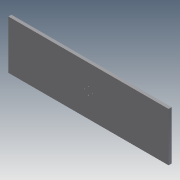
# Autodesk Inventor part: kinect rotate bottom
Saved by Autodesk Inventor 2011 (Build 150239000, 239)
## iProperties
Created: 2012-01-08
Part Number: kinect rotate bottom
Document SubType Name: Modeling
Designer: Matthew
Density: 1 g/cm^3
Author: Matthew
Autodesk Inventor part; units mm, degrees
ref_plane "YZ Plane" through (0, 0, 0) normal (1, 0, 0) x (0, 1, 0)
ref_plane "XZ Plane" through (0, 0, 0) normal (0, 1, 0) x (-1, 0, 0)
ref_plane "XY Plane" through (0, 0, 0) normal (0, 0, 1) x (1, 0, 0)
sketch "Sketch1" plane through (0, 0, 0) normal (0, 0, 1) x (1, 0, 0)
  line L0 (-33.6817, -5.828) -> (300.0743, -5.828)
  line L1 (300.0743, -5.828) -> (300.0743, 7.2749)
  line L2 (300.0743, 7.2749) -> (-33.6817, 7.2749)
  line L3 (-33.6817, 7.2749) -> (-33.6817, -5.828)
  line L4 (-33.6817, 7.2749) -> (300.0743, 7.2749)
  line L5 (300.0743, 7.2749) -> (300.0743, -94.3251)
  line L6 (300.0743, -94.3251) -> (-33.6817, -94.3251)
  line L7 (-33.6817, -94.3251) -> (-33.6817, 7.2749)
  point P0 (0, 0)
  dimension "d0" = 333.756
  dimension "d1" = 101.6
  constraints: 16 end point, 4 parallel, 2 horizontal, 2 perpendicular
  measures "d0" distance of L2.end L1.end
  measures "d1" distance of L4.end L5.end
extrude "Extrusion1" add sketch "Sketch1" along normal blind 6.35
sketch "Sketch2" plane through (0, 0, 6.35) normal (0, 0, 1) x (1, 0, 0)
  circle A0 centre (133.1963, -43.5251) radius 8
  circle A1 centre (133.1963, -35.5251) radius 1
  circle A2 centre (141.1963, -43.5251) radius 1
  circle A3 centre (133.1963, -51.5251) radius 1
  circle A4 centre (125.1963, -43.5251) radius 1
  point P0 (0, 0)
  dimension "d4" = 16
  dimension "d5" = 2
  dimension "d6" = 2
  dimension "d7" = 2
  dimension "d8" = 2
  constraints: 5 centre point, 4 point on circle
  measures "d4" diameter of A0
  measures "d5" diameter of A1
  measures "d6" diameter of A2
  measures "d7" diameter of A3
  measures "d8" diameter of A4
extrude "Extrusion2" cut sketch "Sketch2" against normal blind 6.35 contours A0 A2 | A0 A2 | A1 A0 | A0 A1 | A3 A0 | A0 A3 | A4 A0 | A0 A4
body "Solid1"
